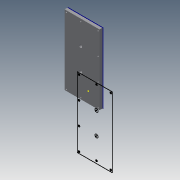
# Autodesk Inventor part: shaft_cover
Saved by Autodesk Inventor 2015 (Build 190159000, 159)
## iProperties
Created: 2014-08-31
Part Number: shaft_cover
Material: Generic
Document SubType Name: Modeling
Designer: shohei
Density: 1 g/cm^3
Appearance: Default
Author: shohei
Autodesk Inventor part; units mm, degrees
ref_plane "YZ Plane" through (0, 0, 0) normal (1, 0, 0) x (0, 1, 0)
ref_plane "XZ Plane" through (0, 0, 0) normal (0, 1, 0) x (-1, 0, 0)
ref_plane "XY Plane" through (0, 0, 0) normal (0, 0, 1) x (1, 0, 0)
sketch "Block1" plane through (0, 0, 0) normal (0, 0, 1) x (1, 0, 0)
  line L0 (-75.22, -185.22) -> (-75.22, 35.22)
  line L1 (-75.22, 35.22) -> (35.22, 35.22)
  line L2 (35.22, 35.22) -> (35.22, -185.22)
  line L3 (35.22, -185.22) -> (-75.22, -185.22)
  circle A0 centre (-70, -180) radius 2.72
  circle A1 centre (-25, -177.5) radius 2.72
  circle A2 centre (30, -180) radius 2.72
  circle A3 centre (-25, 30) radius 2.72
  circle A4 centre (-70, 30) radius 2.72
  circle A5 centre (30, -40) radius 2.72
  circle A6 centre (30, -110) radius 2.72
  circle A7 centre (-25, -110) radius 5.22
  circle A8 centre (-25, -40) radius 5.22
  circle A9 centre (30, 30) radius 2.72
  point P0 (-15, -74.8437)
sketch "Sketch1" plane through (0, 0, 0) normal (0, 1, 0) x (-1, 0, 0)
  line L0 (0, 0) -> (75, 0)
  line L1 (75, 0) -> (75, 185)
  line L2 (75, 185) -> (0, 185)
  circle A0 centre (25, 110) radius 5
  circle A1 centre (25, 40) radius 5
  line L3 (75, 185) -> (100, 185)
  line L4 (75, 0) -> (100, 0)
  line L5 (0, 0) -> (-35, 0)
  line L6 (-35, 0) -> (-35, 185)
  line L7 (-35, 185) -> (0, 185)
  line L8 (106.8257, 75) -> (-45.4509, 75)
  line L9 (-35, 0) -> (75, 0)
  line L10 (75, 0) -> (75, -35)
  line L11 (75, -35) -> (-35, -35)
  line L12 (-35, -35) -> (-35, 0)
  circle A2 centre (-30, 180) radius 2.5
  circle A3 centre (70, 180) radius 2.5
  circle A4 centre (-30, -30) radius 2.5
  circle A5 centre (70, -30) radius 2.5
  circle A6 centre (-30, 110) radius 2.5
  circle A7 centre (-30, 40) radius 2.5
  circle A8 centre (25, 177.5) radius 2.5
  circle A9 centre (25, -30) radius 2.5
  dimension "d5" = 10
  dimension "d9" = 70
  dimension "d13" = 35
  dimension "d14" = 50
  dimension "d17" = 75
  dimension "d18" = 185
  dimension "d19" = 35
  dimension "d22" = 5
  dimension "d23" = 5
  dimension "d24" = 5
  dimension "d25" = 5
  dimension "d26" = 5
  dimension "d27" = 5
  dimension "d28" = 5
  dimension "d29" = 5
  dimension "d30" = 5
  dimension "d31" = 5
  dimension "d32" = 5
  dimension "d33" = 75
  dimension "d34" = 5
  dimension "d35" = 75
  dimension "d36" = 5
  dimension "d37" = 5
  dimension "d38" = 5
  dimension "d39" = 5
  dimension "d42" = 5
  dimension "d43" = 50
  dimension "d46" = 5
  dimension "d47" = 5
  dimension "d48" = 50
  constraints: 26 end point, 10 centre point, 6 horizontal, 4 perpendicular, 3 parallel
  measures "d5" diameter of A0
  measures "d9" distance of A1.centre A0.centre
  measures "d13" distance of L0.start L5.end
  measures "d14" distance from line of A0.centre L1
  measures "d17" distance of L0.start L0.end
  measures "d18" distance of L0.end L1.end
  measures "d19" distance of L9.end L10.end
  measures "d22" diameter of A3
  measures "d23" diameter of A2
  measures "d24" diameter of A6
  measures "d25" diameter of A7
  measures "d26" diameter of A4
  measures "d27" diameter of A5
  measures "d28" distance from line of L2 A3.centre
  measures "d29" distance from line of L7 A2.centre
  measures "d30" distance from line of L6 A2.centre
  measures "d31" distance from line of L1 A3.centre
  measures "d32" distance from line of L6 A6.centre
  measures "d33" distance from line of A6.centre L7
  measures "d34" distance from line of L6 A7.centre
  measures "d35" distance from line of L11 A7.centre
  measures "d36" distance from line of L12 A4.centre
  measures "d37" distance from line of L11 A4.centre
  measures "d38" distance from line of L10 A5.centre
  measures "d39" distance from line of L11 A5.centre
  measures "d42" diameter of A8
  measures "d43" distance from line of L1 A8.centre
  measures "d46" diameter of A9
  measures "d47" distance from line of L11 A9.centre
  measures "d48" distance from line of L10 A9.centre
extrude "Extrusion5" add sketch "Sketch1" along normal blind 10
sketch "Sketch2" plane through (0, 10, 0) normal (0, 1, 0) x (1, 0, 0)
  circle A0 centre (-25, -40) radius 5 projected
  circle A1 centre (-25, -110) radius 5 projected
  circle A2 centre (-25, -177.5) radius 2.5 projected
  circle A3 centre (30, -40) radius 2.5 projected
  circle A4 centre (30, -110) radius 2.5 projected
  circle A5 centre (-70, -180) radius 2.5 projected
  circle A6 centre (30, -180) radius 2.5 projected
  circle A7 centre (-25, 30) radius 2.5 projected
  circle A8 centre (-70, 30) radius 2.5 projected
  circle A9 centre (30, 30) radius 2.5 projected
  line L0 (35, -185) -> (35, 35) projected
  line L1 (35, 35) -> (-75, 35) projected
  line L2 (-75, 35) -> (-75, -185) projected
  line L3 (-75, -185) -> (35, -185) projected
  point P0 (0, 0)
  constraints: 3 perpendicular, 10 other
sketch "DXF" plane through (0, 0, 0) normal (0, 1, 0) x (-1, 0, 0)
  point P0 (0, 0)
body "Solid5"
